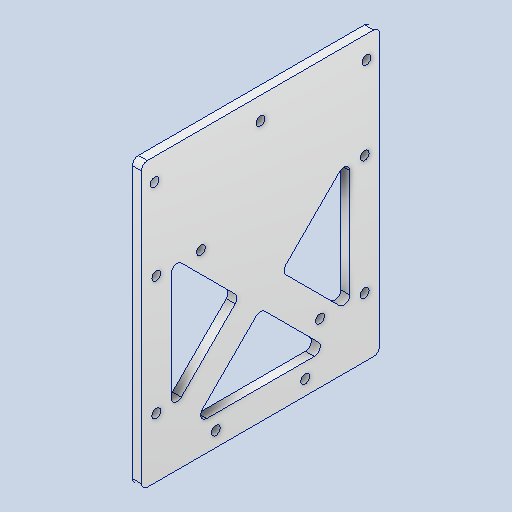
# Autodesk Inventor part: base_weel-v1-Plate-lider-F
Saved by Autodesk Inventor 2025.1 (Build 291241000, 241)
## iProperties
Created: 2024-10-25
Part Number: base_weel-v1-Plate-lider-F
Material: アルミニウム 6061
Document SubType Name: Modeling
Designer: haruy
Density: 2.7 g/cm^3
Appearance: アルミニウム - フラット
Author: haruy
Autodesk Inventor part; units mm, degrees
ref_plane "YZ Plane" through (0, 0, 0) normal (1, 0, 0) x (0, 1, 0)
ref_plane "XZ Plane" through (0, 0, 0) normal (0, 1, 0) x (-1, 0, 0)
ref_plane "XY Plane" through (0, 0, 0) normal (0, 0, 1) x (1, 0, 0)
sketch "スケッチ1" plane through (0, 0, 0) normal (1, 0, 0) x (0, 1, 0)
  line L0 (-149.7065, 436.5093) -> (480.2935, 436.5093)
  line L1 (480.2935, 436.5093) -> (480.2935, -193.4907)
  line L2 (480.2935, -193.4907) -> (-149.7065, -193.4907)
  line L3 (-149.7065, -193.4907) -> (-149.7065, 436.5093)
  line L4 (-149.7065, 436.5093) -> (480.2935, -193.4907) construction
  line L5 (480.2935, 436.5093) -> (-149.7065, -193.4907) construction
  line L6 (-149.7065, 343.7276) -> (-134.7065, 343.7276)
  line L7 (-134.7065, 343.7276) -> (-134.7065, -100.7089)
  line L8 (-134.7065, -100.7089) -> (-149.7065, -100.7089)
  line L9 (-149.7065, -100.7089) -> (-149.7065, 343.7276)
  line L10 (387.5118, 436.5093) -> (-56.9247, 436.5093)
  line L11 (-56.9247, 436.5093) -> (-56.9247, 421.5093)
  line L12 (-56.9247, 421.5093) -> (387.5118, 421.5093)
  line L13 (387.5118, 421.5093) -> (387.5118, 436.5093)
  line L14 (-56.9247, 421.5093) -> (-134.7065, 343.7276)
  line L15 (-134.7065, 343.7276) -> (-134.7065, 436.5093)
  line L16 (-56.9247, 421.5093) -> (-134.7065, 343.7276)
  line L17 (-134.7065, 343.7276) -> (-127.6354, 336.6565)
  line L18 (-127.6354, 336.6565) -> (-49.8537, 414.4382)
  line L19 (-49.8537, 414.4382) -> (-56.9247, 421.5093)
  line L20 (54.5012, 421.5093) -> (-134.7065, 232.3017)
  line L21 (54.5012, 421.5093) -> (-134.7065, 232.3017)
  line L22 (-134.7065, 232.3017) -> (-127.6354, 225.2306)
  line L23 (-127.6354, 225.2306) -> (61.5722, 414.4382)
  line L24 (61.5722, 414.4382) -> (54.5012, 421.5093)
  line L25 (165.2935, 121.5093) -> (-791.3038, 121.5093)
  line L26 (-56.9247, -178.4907) -> (-134.7065, -100.7089)
  line L27 (-134.7065, -100.7089) -> (-127.6354, -93.6379)
  line L28 (-127.6354, -93.6379) -> (-49.8537, -171.4196)
  line L29 (-49.8537, -171.4196) -> (-56.9247, -178.4907)
  line L30 (54.5012, -178.4907) -> (-134.7065, 10.7169)
  line L31 (-134.7065, 10.7169) -> (-127.6354, 17.788)
  line L32 (-127.6354, 17.788) -> (61.5722, -171.4196)
  line L33 (61.5722, -171.4196) -> (54.5012, -178.4907)
  circle A0 centre (165.2935, 121.5093) radius 400
  line L34 (-164.7065, 146.5093) -> (-214.7065, 146.5093)
  line L35 (-214.7065, 146.5093) -> (-214.7065, 96.5093)
  line L36 (-214.7065, 96.5093) -> (-164.7065, 96.5093)
  line L37 (-164.7065, 96.5093) -> (-164.7065, 146.5093)
  line L38 (165.2935, 121.5093) -> (165.2935, -509.4085)
  line L39 (387.5118, 421.5093) -> (465.2935, 343.7276)
  line L40 (465.2935, 343.7276) -> (458.2225, 336.6565)
  line L41 (458.2225, 336.6565) -> (380.4407, 414.4382)
  line L42 (380.4407, 414.4382) -> (387.5118, 421.5093)
  line L43 (276.0859, 421.5093) -> (465.2935, 232.3017)
  line L44 (465.2935, 232.3017) -> (458.2225, 225.2306)
  line L45 (458.2225, 225.2306) -> (269.0148, 414.4382)
  line L46 (269.0148, 414.4382) -> (276.0859, 421.5093)
  line L47 (458.2225, 17.788) -> (269.0148, -171.4196)
  line L48 (465.2935, 10.7169) -> (458.2225, 17.788)
  line L49 (276.0859, -178.4907) -> (465.2935, 10.7169)
  line L50 (269.0148, -171.4196) -> (276.0859, -178.4907)
  line L51 (465.2935, -100.7089) -> (458.2225, -93.6379)
  line L52 (387.5118, -178.4907) -> (465.2935, -100.7089)
  line L53 (458.2225, -93.6379) -> (380.4407, -171.4196)
  line L54 (380.4407, -171.4196) -> (387.5118, -178.4907)
  line L55 (-149.7065, 161.5093) -> (-229.7065, 161.5093)
  line L56 (-229.7065, 161.5093) -> (-229.7065, 151.5093)
  line L57 (-229.7065, 151.5093) -> (-149.7065, 151.5093)
  line L58 (-149.7065, 151.5093) -> (-149.7065, 161.5093)
  line L59 (-229.7065, 151.5093) -> (-219.7065, 151.5093)
  line L60 (-219.7065, 151.5093) -> (-219.7065, 121.5093)
  line L61 (-219.7065, 121.5093) -> (-229.7065, 121.5093)
  line L62 (-229.7065, 121.5093) -> (-229.7065, 151.5093)
  line L63 (465.2935, 343.7276) -> (480.2935, 343.7276)
  line L64 (480.2935, 343.7276) -> (480.2935, -100.7089)
  line L65 (480.2935, -100.7089) -> (465.2935, -100.7089)
  line L66 (465.2935, -100.7089) -> (465.2935, 343.7276)
  line L67 (-56.9247, -193.4907) -> (387.5118, -193.4907)
  line L68 (387.5118, -193.4907) -> (387.5118, -178.4907)
  line L69 (387.5118, -178.4907) -> (-56.9247, -178.4907)
  line L70 (-56.9247, -178.4907) -> (-56.9247, -193.4907)
  line L71 (379.7941, 410.2561) -> (454.0403, 336.0099)
  line L72 (454.0403, 336.0099) -> (419.2302, 301.1998)
  line L73 (419.2302, 301.1998) -> (344.984, 375.446)
  line L74 (344.984, 375.446) -> (379.7941, 410.2561)
  line L75 (480.2935, 436.5093) -> (165.2935, 121.5093)
  line L76 (480.2935, 266.5093) -> (-149.7065, 266.5093)
  line L77 (-149.7065, 266.5093) -> (-149.7065, 246.5093)
  line L78 (-149.7065, 246.5093) -> (480.2935, 246.5093)
  line L79 (480.2935, 246.5093) -> (480.2935, 266.5093)
  line L80 (480.2935, -23.4907) -> (-149.7065, -23.4907)
  line L81 (-149.7065, -3.4907) -> (480.2935, -3.4907)
  line L82 (480.2935, 266.5093) -> (500.2935, 266.5093)
  line L83 (500.2935, 266.5093) -> (500.2935, 286.5093)
  line L84 (500.2935, 286.5093) -> (480.2935, 286.5093)
  line L85 (480.2935, 286.5093) -> (480.2935, 266.5093)
  line L86 (480.2935, -23.4907) -> (500.2935, -23.4907)
  line L87 (500.2935, -23.4907) -> (500.2935, -43.4907)
  line L88 (500.2935, -43.4907) -> (480.2935, -43.4907)
  line L89 (480.2935, -43.4907) -> (480.2935, -23.4907)
  line L90 (500.2935, 286.5093) -> (512.7935, 286.5093)
  line L91 (505.7289, -43.4907) -> (495.7289, -43.4907)
  circle A1 centre (677.2935, 121.5093) radius 122.5
  line L92 (480.2935, 266.5093) -> (500.2935, 266.5093)
  line L93 (500.2935, 266.5093) -> (500.2935, 246.5093)
  line L94 (500.2935, 246.5093) -> (480.2935, 246.5093)
  line L95 (480.2935, 246.5093) -> (480.2935, 266.5093)
  line L96 (480.2935, -23.4907) -> (500.2935, -23.4907)
  line L97 (500.2935, -23.4907) -> (500.2935, -3.4907)
  line L98 (500.2935, -3.4907) -> (480.2935, -3.4907)
  line L99 (480.2935, -3.4907) -> (480.2935, -23.4907)
  line L100 (291.2935, 266.5093) -> (311.2935, 266.5093)
  line L101 (311.2935, 266.5093) -> (311.2935, 286.5093)
  line L102 (311.2935, 286.5093) -> (291.2935, 286.5093)
  line L103 (291.2935, 286.5093) -> (291.2935, 266.5093)
  line L104 (-127.6354, 336.6565) -> (-149.7065, 336.6565)
  circle A2 centre (-142.2065, 353.5093) radius 1.5
  circle A3 centre (-142.2065, 343.5093) radius 1.5
  line L105 (-134.7065, 363.5093) -> (-149.7065, 363.5093)
  line L106 (-56.9247, 429.0093) -> (-142.2065, 429.0093)
  line L107 (-142.2065, 429.0093) -> (-142.2065, 363.5093)
  circle A4 centre (-66.7065, 429.0093) radius 1.5
  circle A5 centre (-56.7065, 429.0093) radius 1.5
  line L108 (-76.7065, 436.5093) -> (-76.7065, 421.5093)
  line L109 (-56.9247, 421.5093) -> (-76.7065, 421.5093)
  circle A6 centre (-66.7065, -185.9907) radius 1.5
  circle A7 centre (-56.7065, -185.9907) radius 1.5
  circle A8 centre (-142.2065, -110.4907) radius 1.5
  circle A9 centre (-142.2065, -100.4907) radius 1.5
  line L110 (-134.7065, -120.4907) -> (-149.7065, -120.4907)
  line L111 (-76.7065, -193.4907) -> (-76.7065, -178.4907)
  line L112 (407.2935, 436.5093) -> (407.2935, 421.5093)
  circle A10 centre (397.2935, 429.0093) radius 1.5
  circle A11 centre (387.2935, 429.0093) radius 1.5
  line L113 (465.2935, 363.5093) -> (480.2935, 363.5093)
  circle A12 centre (472.7935, 353.5093) radius 1.5
  circle A13 centre (472.7935, 343.5093) radius 1.5
  line L114 (465.2935, -120.4907) -> (480.2935, -120.4907)
  circle A14 centre (472.7935, -110.4907) radius 1.5
  circle A15 centre (472.7935, -100.4907) radius 1.5
  line L115 (407.2935, -193.4907) -> (407.2935, -178.4907)
  circle A16 centre (397.2935, -185.9907) radius 1.5
  circle A17 centre (387.2935, -185.9907) radius 1.5
  line L116 (-134.7065, -100.7089) -> (-134.7065, -120.4907)
  line L117 (-56.9247, -178.4907) -> (-76.7065, -178.4907)
  line L118 (407.2935, -178.4907) -> (387.5118, -178.4907)
  line L119 (465.2935, -100.7089) -> (465.2935, -120.4907)
  line L120 (465.2935, 363.5093) -> (465.2935, 343.7276)
  line L121 (387.5118, 421.5093) -> (407.2935, 421.5093)
  circle A18 centre (-127.6354, 343.7276) radius 1.5
  circle A19 centre (-120.5643, 350.7986) radius 1.5
  circle A20 centre (-127.6354, 232.3017) radius 1.5
  circle A21 centre (-120.5643, 239.3728) radius 1.5
  circle A22 centre (-63.9958, 407.3672) radius 1.5
  circle A23 centre (-56.9247, 414.4382) radius 1.5
  circle A24 centre (47.4301, 407.3672) radius 1.5
  circle A25 centre (54.5012, 414.4382) radius 1.5
  circle A26 centre (-56.9247, -171.4196) radius 1.5
  circle A27 centre (-63.9958, -164.3485) radius 1.5
  circle A28 centre (54.5012, -171.4196) radius 1.5
  circle A29 centre (47.4301, -164.3485) radius 1.5
  circle A30 centre (-127.6354, -100.7089) radius 1.5
  circle A31 centre (-120.5643, -107.78) radius 1.5
  circle A32 centre (-120.5643, 3.6459) radius 1.5
  circle A33 centre (-127.6354, 10.7169) radius 1.5
  circle A34 centre (458.2225, 10.7169) radius 1.5
  circle A35 centre (451.1514, 3.6459) radius 1.5
  circle A36 centre (458.2225, -100.7089) radius 1.5
  circle A37 centre (451.1514, -107.78) radius 1.5
  circle A38 centre (394.5828, -164.3485) radius 1.5
  circle A39 centre (387.5118, -171.4196) radius 1.5
  circle A40 centre (283.157, -164.3485) radius 1.5
  circle A41 centre (276.0859, -171.4196) radius 1.5
  circle A42 centre (451.1514, 239.3728) radius 1.5
  circle A43 centre (458.2225, 232.3017) radius 1.5
  circle A44 centre (458.2225, 343.7276) radius 1.5
  circle A45 centre (451.1514, 350.7986) radius 1.5
  circle A46 centre (394.5828, 407.3672) radius 1.5
  circle A47 centre (387.5118, 414.4382) radius 1.5
  circle A48 centre (276.0859, 414.4382) radius 1.5
  circle A49 centre (283.157, 407.3672) radius 1.5
  circle A50 centre (-142.2065, 232.0834) radius 1.5
  circle A51 centre (-142.2065, 242.0834) radius 1.5
  circle A52 centre (44.7194, 429.0093) radius 1.5
  circle A53 centre (54.7194, 429.0093) radius 1.5
  circle A54 centre (-142.2065, 10.9352) radius 1.5
  circle A55 centre (-142.2065, 0.9352) radius 1.5
  circle A56 centre (44.7194, -185.9907) radius 1.5
  circle A57 centre (54.7194, -185.9907) radius 1.5
  circle A58 centre (275.8676, 429.0093) radius 1.5
  circle A59 centre (285.8676, 429.0093) radius 1.5
  circle A60 centre (472.7935, 242.0834) radius 1.5
  circle A61 centre (472.7935, 232.0834) radius 1.5
  circle A62 centre (472.7935, 0.9352) radius 1.5
  circle A63 centre (472.7935, 10.9352) radius 1.5
  circle A64 centre (285.8676, -185.9907) radius 1.5
  circle A65 centre (275.8676, -185.9907) radius 1.5
  circle A66 centre (472.7935, 256.5093) radius 1.5
  circle A67 centre (472.7935, -13.4907) radius 1.5
  circle A68 centre (-142.2065, -13.4907) radius 1.5
  circle A69 centre (-142.2065, 256.5093) radius 1.5
  circle A70 centre (316.2935, 256.5093) radius 1.5
  circle A71 centre (316.2935, -13.4907) radius 1.5
  circle A72 centre (-209.7065, 141.5093) radius 1.5
  line L122 (-189.7065, 146.5093) -> (-189.7065, 96.5093)
  circle A73 centre (-209.7065, 101.5093) radius 1.5
  circle A74 centre (-169.7065, 141.5093) radius 1.5
  circle A75 centre (-169.7065, 101.5093) radius 1.5
  circle A76 centre (-142.2065, 121.5093) radius 1.5
  circle A77 centre (-142.2065, 157.0834) radius 1.5
  circle A78 centre (-169.7065, 156.5093) radius 1.5
  circle A79 centre (-209.7065, 156.5093) radius 1.5
  circle A80 centre (-224.7065, 136.5093) radius 1.5
  circle A81 centre (-224.7065, 106.5093) radius 1.5
  line L123 (-229.7065, 121.5093) -> (-229.7065, 91.5093)
  line L124 (-229.7065, 91.5093) -> (-149.7065, 91.5093)
  line L125 (-219.7065, 91.5093) -> (-219.7065, 121.5093)
  line L126 (-149.7065, 81.5093) -> (-229.7065, 81.5093)
  line L127 (-229.7065, 81.5093) -> (-229.7065, 91.5093)
  circle A82 centre (-209.7065, 86.5093) radius 1.5
  circle A83 centre (-169.7065, 86.5093) radius 1.5
  circle A84 centre (-142.2065, 85.9352) radius 1.5
  circle A85 centre (-189.7065, 121.5093) radius 10
  line L128 (-214.7065, 146.5093) -> (-189.7065, 121.5093)
  line L129 (-218.242, 142.9738) -> (-193.242, 117.9738)
  line L130 (-218.242, 142.9738) -> (-219.7065, 144.4382)
  line L131 (-211.1709, 150.0449) -> (-186.1709, 125.0449)
  line L132 (-211.1709, 150.0449) -> (-212.6354, 151.5093)
  line L133 (-211.1709, 92.9738) -> (-186.1709, 117.9738)
  line L134 (-218.242, 100.0449) -> (-193.242, 125.0449)
  line L135 (-168.242, 150.0449) -> (-193.242, 125.0449)
  line L136 (-168.242, 92.9738) -> (-193.242, 117.9738)
  line L137 (-218.242, 100.0449) -> (-219.7065, 98.5804)
  line L138 (-211.1709, 92.9738) -> (-212.6354, 91.5093)
  line L139 (-168.242, 150.0449) -> (-166.7775, 151.5093)
  line L140 (-168.242, 92.9738) -> (-166.7775, 91.5093)
  line L141 (-149.7065, 161.5093) -> (-134.7065, 161.5093)
  line L142 (-149.7065, 81.5093) -> (-134.7065, 81.5093)
  point P0 (0, 0)
  point P1 (-149.7065, -23.4907)
  point P2 (480.2935, -3.4907)
  point P3 (-149.7065, 266.5093)
  point P4 (480.2935, 246.5093)
  point P5 (-199.3657, 124.0975)
  point P6 (-199.3657, 118.9211)
  point P7 (-192.2947, 111.8501)
  point P8 (-187.1183, 111.8501)
  point P9 (-189.7065, 128.5804)
  point P10 (-189.7065, 114.4382)
  point P11 (-196.7775, 121.5093)
  dimension "d0" = 3
  dimension "d1" = 68
  dimension "d2" = 7.5
  dimension "d3" = 3
  dimension "d4" = 10
  dimension "d5" = 7.5
  dimension "d6" = 10
  dimension "d7" = 3
  dimension "d8" = 3
  dimension "d9" = 10
  dimension "d10" = 68
  dimension "d11" = 7.5
  dimension "d12" = 7.5
  dimension "d13" = 10
  dimension "d14" = 3
  dimension "d15" = 3
  dimension "d16" = 5
  dimension "d17" = 10
  dimension "d18" = 5
  dimension "d19" = 5
  dimension "d20" = 3
  dimension "d21" = 3
  dimension "d22" = 5
  dimension "d23" = 10
  dimension "d24" = 5
  dimension "d25" = 5
  dimension "d26" = 0.2182
  dimension "d27" = 3
  dimension "d28" = 7.5
  dimension "d29" = 0.2182
  dimension "d30" = 3
  dimension "d31" = 10
  dimension "d32" = 7.5
  dimension "d33" = 3
  dimension "d34" = 7.5
  dimension "d35" = 10
  dimension "d36" = 3
  dimension "d37" = 5
  dimension "d38" = 10
  dimension "d39" = 3
  dimension "d40" = 5
  dimension "d41" = 5
  dimension "d42" = 3
  dimension "d43" = 3
  dimension "d44" = 7.5
  dimension "d45" = 7.5
  dimension "d46" = 75
  dimension "d47" = 3
  dimension "d48" = 3
  dimension "d49" = 5
  dimension "d50" = 5
  dimension "d51" = 20
  dimension "d52" = 20
  dimension "d53" = 3
  dimension "d54" = 15
  dimension "d55" = 5
  dimension "d56" = 20
  dimension "d57" = 5
  dimension "d58" = 5
  constraints: 286 end point, 92 symmetric about line, 86 centre point, 9 point on line, 6 midpoint, 6 perpendicular, 4 collinear, 3 horizontal, 2 parallel, 2 vertical, 65 other
  measures "d0" diameter of A2
  measures "d1" distance from line of A2.centre L12
  measures "d2" distance from line of A2.centre L3
  measures "d3" diameter of A3
  measures "d4" distance of A2.centre A3.centre
  measures "d5" distance from line of A3.centre L3
  measures "d6" distance from line of L105 A2.centre
  measures "d7" diameter of A4
  measures "d8" diameter of A5
  measures "d9" distance of A4.centre A5.centre
  measures "d10" horizontal distance of L105.start A4.centre
  measures "d11" distance from line of A4.centre L0
  measures "d12" distance from line of L10 A5.centre
  measures "d13" distance from line of L108 A4.centre
  measures "d14" diameter of A18
  measures "d15" diameter of A19
  measures "d16" distance from line of A18.centre L17
  measures "d17" distance of A19.centre A18.centre
  measures "d18" distance from line of A18.centre L14
  measures "d19" distance from line of A19.centre L14
  measures "d20" diameter of A20
  measures "d21" diameter of A21
  measures "d22" distance from line of A20.centre L22
  measures "d23" distance of A21.centre A20.centre
  measures "d24" distance from line of A20.centre L20
  measures "d25" distance from line of A21.centre L20
  measures "d26" vertical distance of A3.centre A18.centre
  measures "d27" diameter of A50
  measures "d28" distance from line of A50.centre L3
  measures "d29" vertical distance of A50.centre A20.centre
  measures "d30" diameter of A51
  measures "d31" distance of A50.centre A51.centre
  measures "d32" distance from line of L3 A51.centre
  measures "d33" diameter of A66
  measures "d34" distance from line of A66.centre L1
  measures "d35" distance from line of A66.centre L76
  measures "d36" diameter of A70
  measures "d37" distance from line of A70.centre L101
  measures "d38" distance from line of L76 A70.centre
  measures "d39" diameter of A72
  measures "d40" distance from line of A72.centre L35
  measures "d41" distance from line of A72.centre L34
  measures "d42" diameter of A76
  measures "d43" diameter of A77
  measures "d44" distance from line of A76.centre L9
  measures "d45" distance from line of A77.centre L9
  measures "d46" distance of A77.centre A50.centre
  measures "d47" diameter of A78
  measures "d48" diameter of A79
  measures "d49" distance from line of L55 A78.centre
  measures "d50" distance from line of A79.centre L55
  measures "d51" distance from line of A79.centre L56
  measures "d52" distance from line of A78.centre L9
  measures "d53" diameter of A80
  measures "d54" distance from line of A80.centre L59
  measures "d55" distance from line of A80.centre L62
  measures "d56" diameter of A85
  measures "d57" distance between parallel lines of L128 L129
  measures "d58" distance between parallel lines of L128 L131
extrude "押し出し1" add sketch "スケッチ1" against normal blind 3 contours L62 L57 L60 L25 | L25 L125 L124 L123 | L56 L55 L3 L57 | L124 L3 L126 L127 | L60 L57 L132 L131 L34 L35 L129 L130 | L137 L134 L35 L36 L133 L138 L124 L125 | A85 L129 L25 | L25 L134 A85 | L35 L128 A72 A85 L129 | L134 A85 L133 L36 L35 | L141 L7 L25 A76 L3 | L3 L25 A76 L7 L142 | L134 L128 L25 | L25 L122 L136 L129 | L129 L136 L133 A85 L134 | L129 A85 L128 L134 | L34 L131 A85 L128 A72 | L3 L25 L37 L34 L135 L139 L57 | L140 L136 L36 L37 L25 L3 L124 | L122 L135 A85 L25 | L128 L135 L122 | L25 A85 L136 L122 | L128 A85 L131 L135 | L133 L122 A85 | L128 A72 | A72 L128 | A85 L135 L34 L37 L25 | L25 L37 L36 L136 A85 | L136 A85 L122 | A75
extrude "押し出し2" cut sketch "スケッチ1" against normal blind 3 contours A85 L129 L25 | L25 L134 A85 | L133 L122 A85 | L136 A85 L122
fillet "フィレット1" radius 2 13 edges at (-1.5, -229.7065, 161.5093) (-1.5, -229.7065, 81.5093) (-1.5, -196.7775, 121.5093) (-1.5, -219.7065, 144.4382) (-1.5, -219.7065, 98.5804) (-1.5, -189.7065, 114.4382) (-1.5, -166.7775, 91.5093) (-1.5, -212.6354, 91.5093) (-1.5, -166.7775, 151.5093) (-1.5, -189.7065, 128.5804) (-1.5, -212.6354, 151.5093) (-1.5, -134.7065, 161.5093) (-1.5, -134.7065, 81.5093)
equation "\"d5\" = d2"
equation "\"d12\" = d11"
equation "\"d19\" = d18"
equation "\"d25\" = d24"
equation "\"d29\" = d26"
equation "\"d32\" = d28"
equation "\"d45\" = d44"
equation "\"d50\" = d49"
